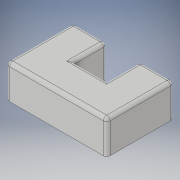
# Autodesk Inventor part: stand_stop
Saved by Autodesk Inventor 2019 (Build 230136000, 136)
## iProperties
Created: 2019-12-27
Part Number: stand_stop
Material: Типовые
Document SubType Name: Modeling
Designer: stepa
Density: 1 g/cm^3
Appearance: По умолчанию
Author: stepa
Autodesk Inventor part; units mm, degrees
ref_plane "YZ Plane" through (0, 0, 0) normal (1, 0, 0) x (0, 1, 0)
ref_plane "XZ Plane" through (0, 0, 0) normal (0, 1, 0) x (-1, 0, 0)
ref_plane "XY Plane" through (0, 0, 0) normal (0, 0, 1) x (1, 0, 0)
sketch "Эскиз1" plane through (0, 0, 0) normal (0, 1, 0) x (-1, 0, 0)
  line L0 (17.4798, -42.1371) -> (-42.5202, -42.1371)
  line L1 (-42.5202, -42.1371) -> (-42.5202, -82.1371)
  line L2 (-42.5202, -82.1371) -> (-22.5202, -82.1371)
  line L3 (-22.5202, -82.1371) -> (-22.5202, -62.1371)
  line L4 (-22.5202, -62.1371) -> (-2.5202, -62.1371)
  line L5 (-2.5202, -62.1371) -> (-2.5202, -82.1371)
  line L6 (-2.5202, -82.1371) -> (17.4798, -82.1371)
  line L7 (17.4798, -82.1371) -> (17.4798, -42.1371)
  point P0 (0, 0)
  dimension "d1" = 40
  dimension "d3" = 20
  dimension "d4" = 20
  dimension "d5" = 20
  constraints: 16 end point, 6 perpendicular, 2 point on line, 1 collinear, 1 horizontal
  measures "d1" distance of L6.end L0.start
  measures "d3" distance between parallel lines of L3 L5
  measures "d4" distance of L5.end L6.end
  measures "d5" distance between parallel lines of L0 L4
extrude "Выдавливание1" add sketch "Эскиз1" along normal blind 20
fillet "Сопряжение1" radius 2 14 edges at (-17.4798, 20, -62.1371) (12.5202, 20, -42.1371) (2.5202, 20, -72.1371) (12.5202, 20, -62.1371) (-7.4798, 20, -82.1371) (22.5202, 20, -72.1371) (32.5202, 20, -82.1371) (42.5202, 20, -62.1371) (42.5202, 10, -82.1371) (2.5202, 10, -82.1371) (22.5202, 10, -82.1371) (-17.4798, 10, -82.1371) (-17.4798, 10, -42.1371) (42.5202, 10, -42.1371)
sketch "Эскиз2" plane through (0, 0, 0) normal (0, -1, 0) x (1, 0, 0)
  line L0 (-15.4798, -42.1371) -> (40.5202, -42.1371) projected
  point P0 (0, 0)
  point P1 (32.9606, -52.1371)
  point P2 (-7.0394, -52.1371)
  dimension "d9" = 40
  dimension "d10" = 10
  constraints: 1 horizontal alignment
  measures "d9" distance of point (-7.039, -52.137) point (32.961, -52.137)
  measures "d10" distance from line of L0 point (32.961, -52.137)
hole "Отверстие1" at (32.9606, 0, -52.1371) at (-7.0394, 0, -52.1371) direction (0, 1, 0) diameter 3 depth 10 tip angle 90
